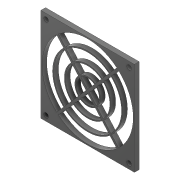
# Autodesk Inventor part: Rejilla Plástica 80 x 80 x 25
Saved by Autodesk Inventor 2020 (Build 240168000, 168)
## iProperties
Created: 2020-09-20
Part Number: Rejilla Plástica 80 x 80 x 25
Material: PPS Plastic
Document SubType Name: Modeling
Designer: Hernan
Density: 1.637 g/cm^3
Appearance: Smooth - White
Author: Hernan
Autodesk Inventor part; units mm, degrees
ref_plane "YZ Plane" through (0, 0, 0) normal (1, 0, 0) x (0, 1, 0)
ref_plane "XZ Plane" through (0, 0, 0) normal (0, 1, 0) x (-1, 0, 0)
ref_plane "XY Plane" through (0, 0, 0) normal (0, 0, 1) x (1, 0, 0)
sketch "Sketch1" plane through (0, 0, 0) normal (0, 0, 1) x (1, 0, 0)
  line L0 (-93.447, 98.412) -> (-13.447, 98.412)
  line L1 (-13.447, 98.412) -> (-13.447, 18.412)
  line L2 (-13.447, 18.412) -> (-93.447, 18.412)
  line L3 (-93.447, 18.412) -> (-93.447, 98.412)
  circle A0 centre (-53.447, 58.412) radius 40.0002
  line L4 (-26.9672, 29.7793) -> (-52.1161, 58.412)
  line L5 (-79.9268, 29.7793) -> (-54.778, 58.412)
  line L6 (-28.4699, 28.4594) -> (-53.447, 56.8967)
  line L7 (-78.4241, 28.4594) -> (-53.447, 56.8967)
  circle A1 centre (-88.947, 93.912) radius 2
  circle A2 centre (-17.947, 93.912) radius 2
  circle A3 centre (-17.947, 22.912) radius 2
  circle A4 centre (-88.947, 22.912) radius 2
  line L8 (-52.1161, 58.412) -> (-40.1746, 72.0077)
  line L9 (-53.447, 59.9274) -> (-41.6773, 73.3276)
  line L10 (-39.5138, 72.7601) -> (-33.5694, 79.5279)
  line L11 (-32.9092, 80.2797) -> (-26.9672, 87.0448)
  line L12 (-41.0165, 74.0799) -> (-35.0721, 80.8478)
  line L13 (-34.4118, 81.5996) -> (-28.4699, 88.3646)
  line L14 (-72.4822, 81.5996) -> (-78.4241, 88.3646)
  line L15 (-73.9849, 80.2797) -> (-79.9268, 87.0448)
  line L16 (-65.8775, 74.0799) -> (-71.8219, 80.8478)
  line L17 (-67.3802, 72.7601) -> (-73.3246, 79.5279)
  line L18 (-53.447, 59.9274) -> (-59.2618, 66.5477)
  line L19 (-59.9247, 67.3024) -> (-65.2167, 73.3276)
  line L20 (-54.778, 58.412) -> (-60.7645, 65.2278)
  line L21 (-61.4274, 65.9826) -> (-66.7194, 72.0077)
  arc A5 (-28.4699, 88.3646) -> (-78.4241, 88.3646) centre (-53.447, 58.412) ccw
  arc A6 (-79.9268, 87.0448) -> (-79.9268, 29.7793) centre (-53.447, 58.412) ccw
  arc A7 (-59.2618, 50.2764) -> (-47.6323, 50.2764) centre (-53.447, 58.412) ccw
  arc A8 (-46.1296, 51.5962) -> (-46.1296, 65.2278) centre (-53.447, 58.412) ccw
  arc A9 (-59.9247, 49.5216) -> (-46.9693, 49.5216) centre (-53.447, 58.412) ccw
  arc A10 (-45.4666, 50.8414) -> (-45.4666, 65.9826) centre (-53.447, 58.412) ccw
  arc A11 (-65.2167, 43.4965) -> (-41.6773, 43.4965) centre (-53.447, 58.412) ccw
  arc A12 (-40.1746, 44.8163) -> (-40.1746, 72.0077) centre (-53.447, 58.412) ccw
  arc A13 (-65.8775, 42.7441) -> (-41.0165, 42.7441) centre (-53.447, 58.412) ccw
  arc A14 (-39.5138, 44.064) -> (-39.5138, 72.7601) centre (-53.447, 58.412) ccw
  arc A15 (-71.8219, 35.9763) -> (-35.0721, 35.9763) centre (-53.447, 58.412) ccw
  arc A16 (-33.5694, 37.2961) -> (-33.5694, 79.5279) centre (-53.447, 58.412) ccw
  arc A17 (-72.4822, 35.2245) -> (-34.4118, 35.2245) centre (-53.447, 58.412) ccw
  arc A18 (-32.9092, 36.5443) -> (-32.9092, 80.2797) centre (-53.447, 58.412) ccw
  arc A19 (-78.4241, 28.4594) -> (-28.4699, 28.4594) centre (-53.447, 58.412) ccw
  arc A20 (-26.9672, 29.7793) -> (-26.9672, 87.0448) centre (-53.447, 58.412) ccw
  arc A21 (-47.6323, 66.5477) -> (-59.2618, 66.5477) centre (-53.447, 58.412) ccw
  arc A22 (-60.7645, 65.2278) -> (-60.7645, 51.5962) centre (-53.447, 58.412) ccw
  arc A23 (-46.9693, 67.3024) -> (-59.9247, 67.3024) centre (-53.447, 58.412) ccw
  arc A24 (-61.4274, 65.9826) -> (-61.4274, 50.8414) centre (-53.447, 58.412) ccw
  arc A25 (-41.6773, 73.3276) -> (-65.2167, 73.3276) centre (-53.447, 58.412) ccw
  arc A26 (-66.7194, 72.0077) -> (-66.7194, 44.8163) centre (-53.447, 58.412) ccw
  arc A27 (-41.0165, 74.0799) -> (-65.8775, 74.0799) centre (-53.447, 58.412) ccw
  arc A28 (-67.3802, 72.7601) -> (-67.3802, 44.064) centre (-53.447, 58.412) ccw
  arc A29 (-35.0721, 80.8478) -> (-71.8219, 80.8478) centre (-53.447, 58.412) ccw
  arc A30 (-73.3246, 79.5279) -> (-73.3246, 37.2961) centre (-53.447, 58.412) ccw
  arc A31 (-34.4118, 81.5996) -> (-72.4822, 81.5996) centre (-53.447, 58.412) ccw
  arc A32 (-73.9849, 80.2797) -> (-73.9849, 36.5443) centre (-53.447, 58.412) ccw
  dimension "d0" = 80
  dimension "d1" = 80
  dimension "d13" = 4
  dimension "d14" = 4
  dimension "d15" = 4
  dimension "d16" = 4
  dimension "d19" = 71
  dimension "d20" = 4.5
  dimension "d21" = 4.5
  dimension "d22" = 71
  dimension "d23" = 4.5
  dimension "d24" = 4.5
  dimension "d25" = 4.5
  dimension "d26" = 4.5
  dimension "d27" = 40
  constraints: 56 point on circle, 44 end point, 33 centre point, 28 point on line, 27 parallel, 7 coincident, 1 horizontal, 1 perpendicular
  measures "d0" distance of L1.end L2.end
  measures "d1" distance of L0.end L1.end
  measures "d13" diameter of A1
  measures "d14" diameter of A2
  measures "d15" diameter of A3
  measures "d16" diameter of A4
  measures "d19" distance of A4.centre A3.centre
  measures "d20" distance from line of A3.centre L1
  measures "d21" distance from line of A2.centre L1
  measures "d22" distance of A1.centre A2.centre
  measures "d23" distance from line of L0 A2.centre
  measures "d24" distance from line of L0 A1.centre
  measures "d25" distance from line of L2 A3.centre
  measures "d26" distance from line of A4.centre L2
  measures "d27" distance from line of L2 A0.centre
extrude "Extrusion1" add sketch "Sketch1" along normal blind 4 contours L0 A0 L3 | L0 L1 A0 | A0 | A0 L2 L3 | L1 L2 A0 | L4 A8 L8 A10 | A17 L7 A15 L6 | A13 L7 A11 L6 | A9 L7 A7 L6
equation "\"d20\" = d25"
equation "\"d21\" = d20"
equation "\"d22\" = d19"
equation "\"d25\" = d23"
body "Solid1"
